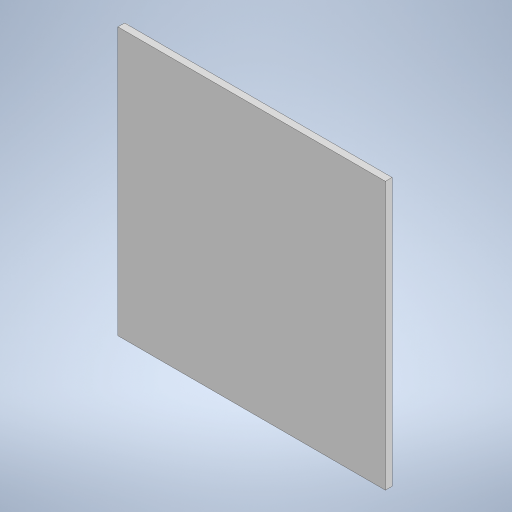
# Autodesk Inventor part: MLAtry1
Saved by Autodesk Inventor 2023 (Build 270158000, 158)
## iProperties
Created: 2022-05-28
Part Number: MLAtry1
Material: Generisch
Document SubType Name: Modeling
Designer: Tim Stechel
Density: 1 g/cm^3
Appearance: Vorgabe
Author: Tim Stechel
Autodesk Inventor part; units mm, degrees
(part 1 of 3)
ref_plane "YZ Plane" through (0, 0, 0) normal (1, 0, 0) x (0, 1, 0)
ref_plane "XZ Plane" through (0, 0, 0) normal (0, 1, 0) x (-1, 0, 0)
ref_plane "XY Plane" through (0, 0, 0) normal (0, 0, 1) x (1, 0, 0)
sketch "Skizze1" plane through (0, 0, 0) normal (0, 0, 1) x (1, 0, 0)
  line L0 (-10, 10) -> (10, 10)
  line L1 (10, 10) -> (10, -10)
  line L2 (10, -10) -> (-10, -10)
  line L3 (-10, -10) -> (-10, 10)
  line L4 (0, -4.8324) -> (0, 6.8811)
  line L5 (-11.9742, 0) -> (8.646, 0)
  line L6 (-10, 10) -> (-10, 9.85)
  line L7 (-10, 9.85) -> (10, 9.85)
  line L8 (-10, 10) -> (-9.85, 10)
  line L9 (-9.85, 10) -> (-9.85, -10)
  circle A0 centre (-9.85, 9.85) radius 0.15
  line L10 (-10, 10) -> (10, 10)
  line L11 (10, 10) -> (10, -10)
  line L12 (10, -10) -> (-10, -10)
  line L13 (-10, -10) -> (-10, 10)
  circle A1 centre (-9.85, 9.55) radius 0.15
  circle A2 centre (-9.85, 9.25) radius 0.15
  circle A3 centre (-9.85, 8.95) radius 0.15
  circle A4 centre (-9.85, 8.65) radius 0.15
  circle A5 centre (-9.85, 8.35) radius 0.15
  circle A6 centre (-9.85, 8.05) radius 0.15
  circle A7 centre (-9.85, 7.75) radius 0.15
  circle A8 centre (-9.85, 7.45) radius 0.15
  circle A9 centre (-9.85, 7.15) radius 0.15
  circle A10 centre (-9.85, 6.85) radius 0.15
  circle A11 centre (-9.85, 6.55) radius 0.15
  circle A12 centre (-9.85, 6.25) radius 0.15
  circle A13 centre (-9.85, 5.95) radius 0.15
  circle A14 centre (-9.85, 5.65) radius 0.15
  circle A15 centre (-9.85, 5.35) radius 0.15
  circle A16 centre (-9.85, 5.05) radius 0.15
  circle A17 centre (-9.85, 4.75) radius 0.15
  circle A18 centre (-9.85, 4.45) radius 0.15
  circle A19 centre (-9.85, 4.15) radius 0.15
  circle A20 centre (-9.85, 3.85) radius 0.15
  circle A21 centre (-9.85, 3.55) radius 0.15
  circle A22 centre (-9.85, 3.25) radius 0.15
  circle A23 centre (-9.85, 2.95) radius 0.15
  circle A24 centre (-9.85, 2.65) radius 0.15
  circle A25 centre (-9.85, 2.35) radius 0.15
  circle A26 centre (-9.85, 2.05) radius 0.15
  circle A27 centre (-9.85, 1.75) radius 0.15
  circle A28 centre (-9.85, 1.45) radius 0.15
  circle A29 centre (-9.85, 1.15) radius 0.15
  circle A30 centre (-9.85, 0.85) radius 0.15
  circle A31 centre (-9.85, 0.55) radius 0.15
  circle A32 centre (-9.85, 0.25) radius 0.15
  circle A33 centre (-9.85, -0.05) radius 0.15
  circle A34 centre (-9.85, -0.35) radius 0.15
  circle A35 centre (-9.85, -0.65) radius 0.15
  circle A36 centre (-9.85, -0.95) radius 0.15
  circle A37 centre (-9.85, -1.25) radius 0.15
  circle A38 centre (-9.85, -1.55) radius 0.15
  circle A39 centre (-9.85, -1.85) radius 0.15
  circle A40 centre (-9.85, -2.15) radius 0.15
  circle A41 centre (-9.85, -2.45) radius 0.15
  circle A42 centre (-9.85, -2.75) radius 0.15
  circle A43 centre (-9.85, -3.05) radius 0.15
  circle A44 centre (-9.85, -3.35) radius 0.15
  circle A45 centre (-9.85, -3.65) radius 0.15
  circle A46 centre (-9.85, -3.95) radius 0.15
  circle A47 centre (-9.85, -4.25) radius 0.15
  circle A48 centre (-9.85, -4.55) radius 0.15
  circle A49 centre (-9.85, -4.85) radius 0.15
  circle A50 centre (-9.55, 9.85) radius 0.15
  circle A51 centre (-9.55, 9.55) radius 0.15
  circle A52 centre (-9.55, 9.25) radius 0.15
  circle A53 centre (-9.55, 8.95) radius 0.15
  circle A54 centre (-9.55, 8.65) radius 0.15
  circle A55 centre (-9.55, 8.35) radius 0.15
  circle A56 centre (-9.55, 8.05) radius 0.15
  circle A57 centre (-9.55, 7.75) radius 0.15
  circle A58 centre (-9.55, 7.45) radius 0.15
  circle A59 centre (-9.55, 7.15) radius 0.15
  circle A60 centre (-9.55, 6.85) radius 0.15
  circle A61 centre (-9.55, 6.55) radius 0.15
  circle A62 centre (-9.55, 6.25) radius 0.15
  circle A63 centre (-9.55, 5.95) radius 0.15
  circle A64 centre (-9.55, 5.65) radius 0.15
  circle A65 centre (-9.55, 5.35) radius 0.15
  circle A66 centre (-9.55, 5.05) radius 0.15
  circle A67 centre (-9.55, 4.75) radius 0.15
  circle A68 centre (-9.55, 4.45) radius 0.15
  circle A69 centre (-9.55, 4.15) radius 0.15
  circle A70 centre (-9.55, 3.85) radius 0.15
  circle A71 centre (-9.55, 3.55) radius 0.15
  circle A72 centre (-9.55, 3.25) radius 0.15
  circle A73 centre (-9.55, 2.95) radius 0.15
  circle A74 centre (-9.55, 2.65) radius 0.15
  circle A75 centre (-9.55, 2.35) radius 0.15
  circle A76 centre (-9.55, 2.05) radius 0.15
  circle A77 centre (-9.55, 1.75) radius 0.15
  circle A78 centre (-9.55, 1.45) radius 0.15
  circle A79 centre (-9.55, 1.15) radius 0.15
  circle A80 centre (-9.55, 0.85) radius 0.15
  circle A81 centre (-9.55, 0.55) radius 0.15
  circle A82 centre (-9.55, 0.25) radius 0.15
  circle A83 centre (-9.55, -0.05) radius 0.15
  circle A84 centre (-9.55, -0.35) radius 0.15
  circle A85 centre (-9.55, -0.65) radius 0.15
  circle A86 centre (-9.55, -0.95) radius 0.15
  circle A87 centre (-9.55, -1.25) radius 0.15
  circle A88 centre (-9.55, -1.55) radius 0.15
  circle A89 centre (-9.55, -1.85) radius 0.15
  circle A90 centre (-9.55, -2.15) radius 0.15
  circle A91 centre (-9.55, -2.45) radius 0.15
  circle A92 centre (-9.55, -2.75) radius 0.15
  circle A93 centre (-9.55, -3.05) radius 0.15
  circle A94 centre (-9.55, -3.35) radius 0.15
  circle A95 centre (-9.55, -3.65) radius 0.15
  circle A96 centre (-9.55, -3.95) radius 0.15
  circle A97 centre (-9.55, -4.25) radius 0.15
  circle A98 centre (-9.55, -4.55) radius 0.15
  circle A99 centre (-9.55, -4.85) radius 0.15
  circle A100 centre (-9.25, 9.85) radius 0.15
  circle A101 centre (-9.25, 9.55) radius 0.15
  circle A102 centre (-9.25, 9.25) radius 0.15
  circle A103 centre (-9.25, 8.95) radius 0.15
  circle A104 centre (-9.25, 8.65) radius 0.15
  circle A105 centre (-9.25, 8.35) radius 0.15
  circle A106 centre (-9.25, 8.05) radius 0.15
  circle A107 centre (-9.25, 7.75) radius 0.15
  circle A108 centre (-9.25, 7.45) radius 0.15
  circle A109 centre (-9.25, 7.15) radius 0.15
  circle A110 centre (-9.25, 6.85) radius 0.15
  circle A111 centre (-9.25, 6.55) radius 0.15
  circle A112 centre (-9.25, 6.25) radius 0.15
  circle A113 centre (-9.25, 5.95) radius 0.15
  circle A114 centre (-9.25, 5.65) radius 0.15
  circle A115 centre (-9.25, 5.35) radius 0.15
  circle A116 centre (-9.25, 5.05) radius 0.15
  circle A117 centre (-9.25, 4.75) radius 0.15
  circle A118 centre (-9.25, 4.45) radius 0.15
  circle A119 centre (-9.25, 4.15) radius 0.15
  circle A120 centre (-9.25, 3.85) radius 0.15
  circle A121 centre (-9.25, 3.55) radius 0.15
  circle A122 centre (-9.25, 3.25) radius 0.15
  circle A123 centre (-9.25, 2.95) radius 0.15
  circle A124 centre (-9.25, 2.65) radius 0.15
  circle A125 centre (-9.25, 2.35) radius 0.15
  circle A126 centre (-9.25, 2.05) radius 0.15
  circle A127 centre (-9.25, 1.75) radius 0.15
  circle A128 centre (-9.25, 1.45) radius 0.15
  circle A129 centre (-9.25, 1.15) radius 0.15
  circle A130 centre (-9.25, 0.85) radius 0.15
  circle A131 centre (-9.25, 0.55) radius 0.15
  circle A132 centre (-9.25, 0.25) radius 0.15
  circle A133 centre (-9.25, -0.05) radius 0.15
  circle A134 centre (-9.25, -0.35) radius 0.15
  circle A135 centre (-9.25, -0.65) radius 0.15
  circle A136 centre (-9.25, -0.95) radius 0.15
  circle A137 centre (-9.25, -1.25) radius 0.15
  circle A138 centre (-9.25, -1.55) radius 0.15
  circle A139 centre (-9.25, -1.85) radius 0.15
  circle A140 centre (-9.25, -2.15) radius 0.15
  circle A141 centre (-9.25, -2.45) radius 0.15
  circle A142 centre (-9.25, -2.75) radius 0.15
  circle A143 centre (-9.25, -3.05) radius 0.15
  circle A144 centre (-9.25, -3.35) radius 0.15
  circle A145 centre (-9.25, -3.65) radius 0.15
  circle A146 centre (-9.25, -3.95) radius 0.15
  circle A147 centre (-9.25, -4.25) radius 0.15
  circle A148 centre (-9.25, -4.55) radius 0.15
  circle A149 centre (-9.25, -4.85) radius 0.15
  circle A150 centre (-8.95, 9.85) radius 0.15
  circle A151 centre (-8.95, 9.55) radius 0.15
  circle A152 centre (-8.95, 9.25) radius 0.15
  circle A153 centre (-8.95, 8.95) radius 0.15
  circle A154 centre (-8.95, 8.65) radius 0.15
  circle A155 centre (-8.95, 8.35) radius 0.15
  circle A156 centre (-8.95, 8.05) radius 0.15
  circle A157 centre (-8.95, 7.75) radius 0.15
  circle A158 centre (-8.95, 7.45) radius 0.15
  circle A159 centre (-8.95, 7.15) radius 0.15
  circle A160 centre (-8.95, 6.85) radius 0.15
  circle A161 centre (-8.95, 6.55) radius 0.15
  circle A162 centre (-8.95, 6.25) radius 0.15
  circle A163 centre (-8.95, 5.95) radius 0.15
  circle A164 centre (-8.95, 5.65) radius 0.15
  circle A165 centre (-8.95, 5.35) radius 0.15
  circle A166 centre (-8.95, 5.05) radius 0.15
  circle A167 centre (-8.95, 4.75) radius 0.15
  circle A168 centre (-8.95, 4.45) radius 0.15
  circle A169 centre (-8.95, 4.15) radius 0.15
  circle A170 centre (-8.95, 3.85) radius 0.15
  circle A171 centre (-8.95, 3.55) radius 0.15
  circle A172 centre (-8.95, 3.25) radius 0.15
  circle A173 centre (-8.95, 2.95) radius 0.15
  circle A174 centre (-8.95, 2.65) radius 0.15
  circle A175 centre (-8.95, 2.35) radius 0.15
  circle A176 centre (-8.95, 2.05) radius 0.15
  circle A177 centre (-8.95, 1.75) radius 0.15
  circle A178 centre (-8.95, 1.45) radius 0.15
  circle A179 centre (-8.95, 1.15) radius 0.15
  circle A180 centre (-8.95, 0.85) radius 0.15
  circle A181 centre (-8.95, 0.55) radius 0.15
  circle A182 centre (-8.95, 0.25) radius 0.15
  circle A183 centre (-8.95, -0.05) radius 0.15
  circle A184 centre (-8.95, -0.35) radius 0.15
  circle A185 centre (-8.95, -0.65) radius 0.15
  circle A186 centre (-8.95, -0.95) radius 0.15
  circle A187 centre (-8.95, -1.25) radius 0.15
  circle A188 centre (-8.95, -1.55) radius 0.15
  circle A189 centre (-8.95, -1.85) radius 0.15
  circle A190 centre (-8.95, -2.15) radius 0.15
  circle A191 centre (-8.95, -2.45) radius 0.15
  circle A192 centre (-8.95, -2.75) radius 0.15
  circle A193 centre (-8.95, -3.05) radius 0.15
  circle A194 centre (-8.95, -3.35) radius 0.15
  circle A195 centre (-8.95, -3.65) radius 0.15
  circle A196 centre (-8.95, -3.95) radius 0.15
  circle A197 centre (-8.95, -4.25) radius 0.15
  circle A198 centre (-8.95, -4.55) radius 0.15
  circle A199 centre (-8.95, -4.85) radius 0.15
  circle A200 centre (-8.65, 9.85) radius 0.15
  circle A201 centre (-8.65, 9.55) radius 0.15
  circle A202 centre (-8.65, 9.25) radius 0.15
  circle A203 centre (-8.65, 8.95) radius 0.15
  circle A204 centre (-8.65, 8.65) radius 0.15
  circle A205 centre (-8.65, 8.35) radius 0.15
  circle A206 centre (-8.65, 8.05) radius 0.15
  circle A207 centre (-8.65, 7.75) radius 0.15
  circle A208 centre (-8.65, 7.45) radius 0.15
  circle A209 centre (-8.65, 7.15) radius 0.15
  circle A210 centre (-8.65, 6.85) radius 0.15
  circle A211 centre (-8.65, 6.55) radius 0.15
  circle A212 centre (-8.65, 6.25) radius 0.15
  circle A213 centre (-8.65, 5.95) radius 0.15
  circle A214 centre (-8.65, 5.65) radius 0.15
  circle A215 centre (-8.65, 5.35) radius 0.15
  circle A216 centre (-8.65, 5.05) radius 0.15
  circle A217 centre (-8.65, 4.75) radius 0.15
  circle A218 centre (-8.65, 4.45) radius 0.15
  circle A219 centre (-8.65, 4.15) radius 0.15
  circle A220 centre (-8.65, 3.85) radius 0.15
  circle A221 centre (-8.65, 3.55) radius 0.15
  circle A222 centre (-8.65, 3.25) radius 0.15
  circle A223 centre (-8.65, 2.95) radius 0.15
  circle A224 centre (-8.65, 2.65) radius 0.15
  circle A225 centre (-8.65, 2.35) radius 0.15
  circle A226 centre (-8.65, 2.05) radius 0.15
  circle A227 centre (-8.65, 1.75) radius 0.15
  circle A228 centre (-8.65, 1.45) radius 0.15
  circle A229 centre (-8.65, 1.15) radius 0.15
  circle A230 centre (-8.65, 0.85) radius 0.15
  circle A231 centre (-8.65, 0.55) radius 0.15
  circle A232 centre (-8.65, 0.25) radius 0.15
  circle A233 centre (-8.65, -0.05) radius 0.15
  circle A234 centre (-8.65, -0.35) radius 0.15
  circle A235 centre (-8.65, -0.65) radius 0.15
  circle A236 centre (-8.65, -0.95) radius 0.15
  circle A237 centre (-8.65, -1.25) radius 0.15
  circle A238 centre (-8.65, -1.55) radius 0.15
  circle A239 centre (-8.65, -1.85) radius 0.15
  circle A240 centre (-8.65, -2.15) radius 0.15
  circle A241 centre (-8.65, -2.45) radius 0.15
  circle A242 centre (-8.65, -2.75) radius 0.15
  circle A243 centre (-8.65, -3.05) radius 0.15
  circle A244 centre (-8.65, -3.35) radius 0.15
  circle A245 centre (-8.65, -3.65) radius 0.15
  circle A246 centre (-8.65, -3.95) radius 0.15
  circle A247 centre (-8.65, -4.25) radius 0.15
  circle A248 centre (-8.65, -4.55) radius 0.15
  circle A249 centre (-8.65, -4.85) radius 0.15
  circle A250 centre (-8.35, 9.85) radius 0.15
  circle A251 centre (-8.35, 9.55) radius 0.15
  circle A252 centre (-8.35, 9.25) radius 0.15
  circle A253 centre (-8.35, 8.95) radius 0.15
  circle A254 centre (-8.35, 8.65) radius 0.15
  circle A255 centre (-8.35, 8.35) radius 0.15
  circle A256 centre (-8.35, 8.05) radius 0.15
  circle A257 centre (-8.35, 7.75) radius 0.15
  circle A258 centre (-8.35, 7.45) radius 0.15
  circle A259 centre (-8.35, 7.15) radius 0.15
  circle A260 centre (-8.35, 6.85) radius 0.15
  circle A261 centre (-8.35, 6.55) radius 0.15
  circle A262 centre (-8.35, 6.25) radius 0.15
  circle A263 centre (-8.35, 5.95) radius 0.15
  circle A264 centre (-8.35, 5.65) radius 0.15
  circle A265 centre (-8.35, 5.35) radius 0.15
  circle A266 centre (-8.35, 5.05) radius 0.15
  circle A267 centre (-8.35, 4.75) radius 0.15
  circle A268 centre (-8.35, 4.45) radius 0.15
  circle A269 centre (-8.35, 4.15) radius 0.15
  circle A270 centre (-8.35, 3.85) radius 0.15
  circle A271 centre (-8.35, 3.55) radius 0.15
  circle A272 centre (-8.35, 3.25) radius 0.15
  circle A273 centre (-8.35, 2.95) radius 0.15
  circle A274 centre (-8.35, 2.65) radius 0.15
  circle A275 centre (-8.35, 2.35) radius 0.15
  circle A276 centre (-8.35, 2.05) radius 0.15
  circle A277 centre (-8.35, 1.75) radius 0.15
  circle A278 centre (-8.35, 1.45) radius 0.15
  circle A279 centre (-8.35, 1.15) radius 0.15
  circle A280 centre (-8.35, 0.85) radius 0.15
  circle A281 centre (-8.35, 0.55) radius 0.15
  circle A282 centre (-8.35, 0.25) radius 0.15
  circle A283 centre (-8.35, -0.05) radius 0.15
  circle A284 centre (-8.35, -0.35) radius 0.15
  circle A285 centre (-8.35, -0.65) radius 0.15
  circle A286 centre (-8.35, -0.95) radius 0.15
  circle A287 centre (-8.35, -1.25) radius 0.15
  circle A288 centre (-8.35, -1.55) radius 0.15
  circle A289 centre (-8.35, -1.85) radius 0.15
  circle A290 centre (-8.35, -2.15) radius 0.15
  circle A291 centre (-8.35, -2.45) radius 0.15
  circle A292 centre (-8.35, -2.75) radius 0.15
  circle A293 centre (-8.35, -3.05) radius 0.15
  circle A294 centre (-8.35, -3.35) radius 0.15
  circle A295 centre (-8.35, -3.65) radius 0.15
  circle A296 centre (-8.35, -3.95) radius 0.15
  circle A297 centre (-8.35, -4.25) radius 0.15
  circle A298 centre (-8.35, -4.55) radius 0.15
  circle A299 centre (-8.35, -4.85) radius 0.15
  circle A300 centre (-8.05, 9.85) radius 0.15
  circle A301 centre (-8.05, 9.55) radius 0.15
  circle A302 centre (-8.05, 9.25) radius 0.15
  circle A303 centre (-8.05, 8.95) radius 0.15
  circle A304 centre (-8.05, 8.65) radius 0.15
  circle A305 centre (-8.05, 8.35) radius 0.15
  circle A306 centre (-8.05, 8.05) radius 0.15
  circle A307 centre (-8.05, 7.75) radius 0.15
  circle A308 centre (-8.05, 7.45) radius 0.15
  circle A309 centre (-8.05, 7.15) radius 0.15
  circle A310 centre (-8.05, 6.85) radius 0.15
  circle A311 centre (-8.05, 6.55) radius 0.15
  circle A312 centre (-8.05, 6.25) radius 0.15
  circle A313 centre (-8.05, 5.95) radius 0.15
  circle A314 centre (-8.05, 5.65) radius 0.15
  circle A315 centre (-8.05, 5.35) radius 0.15
  circle A316 centre (-8.05, 5.05) radius 0.15
  circle A317 centre (-8.05, 4.75) radius 0.15
  circle A318 centre (-8.05, 4.45) radius 0.15
  circle A319 centre (-8.05, 4.15) radius 0.15
  circle A320 centre (-8.05, 3.85) radius 0.15
  circle A321 centre (-8.05, 3.55) radius 0.15
  circle A322 centre (-8.05, 3.25) radius 0.15
  circle A323 centre (-8.05, 2.95) radius 0.15
  circle A324 centre (-8.05, 2.65) radius 0.15
  circle A325 centre (-8.05, 2.35) radius 0.15
  circle A326 centre (-8.05, 2.05) radius 0.15
  circle A327 centre (-8.05, 1.75) radius 0.15
  circle A328 centre (-8.05, 1.45) radius 0.15
  circle A329 centre (-8.05, 1.15) radius 0.15
  circle A330 centre (-8.05, 0.85) radius 0.15
  circle A331 centre (-8.05, 0.55) radius 0.15
  circle A332 centre (-8.05, 0.25) radius 0.15
  circle A333 centre (-8.05, -0.05) radius 0.15
  circle A334 centre (-8.05, -0.35) radius 0.15
  circle A335 centre (-8.05, -0.65) radius 0.15
  circle A336 centre (-8.05, -0.95) radius 0.15
  circle A337 centre (-8.05, -1.25) radius 0.15
  circle A338 centre (-8.05, -1.55) radius 0.15
  circle A339 centre (-8.05, -1.85) radius 0.15
  circle A340 centre (-8.05, -2.15) radius 0.15
  circle A341 centre (-8.05, -2.45) radius 0.15
  circle A342 centre (-8.05, -2.75) radius 0.15
  circle A343 centre (-8.05, -3.05) radius 0.15
  circle A344 centre (-8.05, -3.35) radius 0.15
  circle A345 centre (-8.05, -3.65) radius 0.15
  circle A346 centre (-8.05, -3.95) radius 0.15
  circle A347 centre (-8.05, -4.25) radius 0.15
  circle A348 centre (-8.05, -4.55) radius 0.15
  circle A349 centre (-8.05, -4.85) radius 0.15
  circle A350 centre (-7.75, 9.85) radius 0.15
  circle A351 centre (-7.75, 9.55) radius 0.15
  circle A352 centre (-7.75, 9.25) radius 0.15
  circle A353 centre (-7.75, 8.95) radius 0.15
  circle A354 centre (-7.75, 8.65) radius 0.15
  circle A355 centre (-7.75, 8.35) radius 0.15
  circle A356 centre (-7.75, 8.05) radius 0.15
  circle A357 centre (-7.75, 7.75) radius 0.15
  circle A358 centre (-7.75, 7.45) radius 0.15
  circle A359 centre (-7.75, 7.15) radius 0.15
  circle A360 centre (-7.75, 6.85) radius 0.15
  circle A361 centre (-7.75, 6.55) radius 0.15
  circle A362 centre (-7.75, 6.25) radius 0.15
  circle A363 centre (-7.75, 5.95) radius 0.15
  circle A364 centre (-7.75, 5.65) radius 0.15
  circle A365 centre (-7.75, 5.35) radius 0.15
  circle A366 centre (-7.75, 5.05) radius 0.15
  circle A367 centre (-7.75, 4.75) radius 0.15
  circle A368 centre (-7.75, 4.45) radius 0.15
  circle A369 centre (-7.75, 4.15) radius 0.15
  circle A370 centre (-7.75, 3.85) radius 0.15
  circle A371 centre (-7.75, 3.55) radius 0.15
  circle A372 centre (-7.75, 3.25) radius 0.15
  circle A373 centre (-7.75, 2.95) radius 0.15
  circle A374 centre (-7.75, 2.65) radius 0.15
  circle A375 centre (-7.75, 2.35) radius 0.15
  circle A376 centre (-7.75, 2.05) radius 0.15
  circle A377 centre (-7.75, 1.75) radius 0.15
  circle A378 centre (-7.75, 1.45) radius 0.15
  circle A379 centre (-7.75, 1.15) radius 0.15
  circle A380 centre (-7.75, 0.85) radius 0.15
  circle A381 centre (-7.75, 0.55) radius 0.15
  circle A382 centre (-7.75, 0.25) radius 0.15
  circle A383 centre (-7.75, -0.05) radius 0.15
  circle A384 centre (-7.75, -0.35) radius 0.15
  circle A385 centre (-7.75, -0.65) radius 0.15
  circle A386 centre (-7.75, -0.95) radius 0.15
  circle A387 centre (-7.75, -1.25) radius 0.15
  circle A388 centre (-7.75, -1.55) radius 0.15
  circle A389 centre (-7.75, -1.85) radius 0.15
  circle A390 centre (-7.75, -2.15) radius 0.15
  circle A391 centre (-7.75, -2.45) radius 0.15
  circle A392 centre (-7.75, -2.75) radius 0.15
  circle A393 centre (-7.75, -3.05) radius 0.15
  circle A394 centre (-7.75, -3.35) radius 0.15
  circle A395 centre (-7.75, -3.65) radius 0.15
  circle A396 centre (-7.75, -3.95) radius 0.15
  circle A397 centre (-7.75, -4.25) radius 0.15
  circle A398 centre (-7.75, -4.55) radius 0.15
  circle A399 centre (-7.75, -4.85) radius 0.15
  circle A400 centre (-7.45, 9.85) radius 0.15
  circle A401 centre (-7.45, 9.55) radius 0.15
  circle A402 centre (-7.45, 9.25) radius 0.15
  circle A403 centre (-7.45, 8.95) radius 0.15
  circle A404 centre (-7.45, 8.65) radius 0.15
  circle A405 centre (-7.45, 8.35) radius 0.15
  circle A406 centre (-7.45, 8.05) radius 0.15
  circle A407 centre (-7.45, 7.75) radius 0.15
  circle A408 centre (-7.45, 7.45) radius 0.15
  circle A409 centre (-7.45, 7.15) radius 0.15
  circle A410 centre (-7.45, 6.85) radius 0.15
  circle A411 centre (-7.45, 6.55) radius 0.15
  circle A412 centre (-7.45, 6.25) radius 0.15
  circle A413 centre (-7.45, 5.95) radius 0.15
  circle A414 centre (-7.45, 5.65) radius 0.15
  circle A415 centre (-7.45, 5.35) radius 0.15
  circle A416 centre (-7.45, 5.05) radius 0.15
  circle A417 centre (-7.45, 4.75) radius 0.15
  circle A418 centre (-7.45, 4.45) radius 0.15
  circle A419 centre (-7.45, 4.15) radius 0.15
  circle A420 centre (-7.45, 3.85) radius 0.15
  circle A421 centre (-7.45, 3.55) radius 0.15
  circle A422 centre (-7.45, 3.25) radius 0.15
  circle A423 centre (-7.45, 2.95) radius 0.15
  circle A424 centre (-7.45, 2.65) radius 0.15
  circle A425 centre (-7.45, 2.35) radius 0.15
  circle A426 centre (-7.45, 2.05) radius 0.15
  circle A427 centre (-7.45, 1.75) radius 0.15
  circle A428 centre (-7.45, 1.45) radius 0.15
  circle A429 centre (-7.45, 1.15) radius 0.15
  circle A430 centre (-7.45, 0.85) radius 0.15
  circle A431 centre (-7.45, 0.55) radius 0.15
  circle A432 centre (-7.45, 0.25) radius 0.15
  circle A433 centre (-7.45, -0.05) radius 0.15
  circle A434 centre (-7.45, -0.35) radius 0.15
  circle A435 centre (-7.45, -0.65) radius 0.15
  circle A436 centre (-7.45, -0.95) radius 0.15
  circle A437 centre (-7.45, -1.25) radius 0.15
  circle A438 centre (-7.45, -1.55) radius 0.15
  circle A439 centre (-7.45, -1.85) radius 0.15
  circle A440 centre (-7.45, -2.15) radius 0.15
  circle A441 centre (-7.45, -2.45) radius 0.15
  circle A442 centre (-7.45, -2.75) radius 0.15
  circle A443 centre (-7.45, -3.05) radius 0.15
  circle A444 centre (-7.45, -3.35) radius 0.15
  circle A445 centre (-7.45, -3.65) radius 0.15
  circle A446 centre (-7.45, -3.95) radius 0.15
  circle A447 centre (-7.45, -4.25) radius 0.15
  circle A448 centre (-7.45, -4.55) radius 0.15
  circle A449 centre (-7.45, -4.85) radius 0.15
  circle A450 centre (-7.15, 9.85) radius 0.15
  circle A451 centre (-7.15, 9.55) radius 0.15
  circle A452 centre (-7.15, 9.25) radius 0.15
  circle A453 centre (-7.15, 8.95) radius 0.15
  circle A454 centre (-7.15, 8.65) radius 0.15
  circle A455 centre (-7.15, 8.35) radius 0.15
  circle A456 centre (-7.15, 8.05) radius 0.15
  circle A457 centre (-7.15, 7.75) radius 0.15
  circle A458 centre (-7.15, 7.45) radius 0.15
  circle A459 centre (-7.15, 7.15) radius 0.15
  circle A460 centre (-7.15, 6.85) radius 0.15
  circle A461 centre (-7.15, 6.55) radius 0.15
  circle A462 centre (-7.15, 6.25) radius 0.15
  circle A463 centre (-7.15, 5.95) radius 0.15
  circle A464 centre (-7.15, 5.65) radius 0.15
  circle A465 centre (-7.15, 5.35) radius 0.15
  circle A466 centre (-7.15, 5.05) radius 0.15
  circle A467 centre (-7.15, 4.75) radius 0.15
  circle A468 centre (-7.15, 4.45) radius 0.15
  circle A469 centre (-7.15, 4.15) radius 0.15
  circle A470 centre (-7.15, 3.85) radius 0.15
  circle A471 centre (-7.15, 3.55) radius 0.15
  circle A472 centre (-7.15, 3.25) radius 0.15
  circle A473 centre (-7.15, 2.95) radius 0.15
  circle A474 centre (-7.15, 2.65) radius 0.15
  circle A475 centre (-7.15, 2.35) radius 0.15
  circle A476 centre (-7.15, 2.05) radius 0.15
  circle A477 centre (-7.15, 1.75) radius 0.15
  circle A478 centre (-7.15, 1.45) radius 0.15
  circle A479 centre (-7.15, 1.15) radius 0.15
  circle A480 centre (-7.15, 0.85) radius 0.15
  circle A481 centre (-7.15, 0.55) radius 0.15
  circle A482 centre (-7.15, 0.25) radius 0.15
  circle A483 centre (-7.15, -0.05) radius 0.15
  circle A484 centre (-7.15, -0.35) radius 0.15
  circle A485 centre (-7.15, -0.65) radius 0.15
  circle A486 centre (-7.15, -0.95) radius 0.15
  circle A487 centre (-7.15, -1.25) radius 0.15
  circle A488 centre (-7.15, -1.55) radius 0.15
  circle A489 centre (-7.15, -1.85) radius 0.15
  circle A490 centre (-7.15, -2.15) radius 0.15
  circle A491 centre (-7.15, -2.45) radius 0.15
  circle A492 centre (-7.15, -2.75) radius 0.15
  circle A493 centre (-7.15, -3.05) radius 0.15
  circle A494 centre (-7.15, -3.35) radius 0.15
  circle A495 centre (-7.15, -3.65) radius 0.15
  circle A496 centre (-7.15, -3.95) radius 0.15
  circle A497 centre (-7.15, -4.25) radius 0.15
  circle A498 centre (-7.15, -4.55) radius 0.15
  circle A499 centre (-7.15, -4.85) radius 0.15
  circle A500 centre (-6.85, 9.85) radius 0.15
  circle A501 centre (-6.85, 9.55) radius 0.15
  circle A502 centre (-6.85, 9.25) radius 0.15
  circle A503 centre (-6.85, 8.95) radius 0.15
  circle A504 centre (-6.85, 8.65) radius 0.15
  circle A505 centre (-6.85, 8.35) radius 0.15
  circle A506 centre (-6.85, 8.05) radius 0.15
  circle A507 centre (-6.85, 7.75) radius 0.15
  circle A508 centre (-6.85, 7.45) radius 0.15
  circle A509 centre (-6.85, 7.15) radius 0.15
  circle A510 centre (-6.85, 6.85) radius 0.15
  circle A511 centre (-6.85, 6.55) radius 0.15
  circle A512 centre (-6.85, 6.25) radius 0.15
  circle A513 centre (-6.85, 5.95) radius 0.15
  circle A514 centre (-6.85, 5.65) radius 0.15
  circle A515 centre (-6.85, 5.35) radius 0.15
  circle A516 centre (-6.85, 5.05) radius 0.15
  circle A517 centre (-6.85, 4.75) radius 0.15
  circle A518 centre (-6.85, 4.45) radius 0.15
  circle A519 centre (-6.85, 4.15) radius 0.15
  circle A520 centre (-6.85, 3.85) radius 0.15
  circle A521 centre (-6.85, 3.55) radius 0.15
  circle A522 centre (-6.85, 3.25) radius 0.15
  circle A523 centre (-6.85, 2.95) radius 0.15
  circle A524 centre (-6.85, 2.65) radius 0.15
  circle A525 centre (-6.85, 2.35) radius 0.15
  circle A526 centre (-6.85, 2.05) radius 0.15
  circle A527 centre (-6.85, 1.75) radius 0.15
  circle A528 centre (-6.85, 1.45) radius 0.15
  circle A529 centre (-6.85, 1.15) radius 0.15
  circle A530 centre (-6.85, 0.85) radius 0.15
  circle A531 centre (-6.85, 0.55) radius 0.15
  circle A532 centre (-6.85, 0.25) radius 0.15
  circle A533 centre (-6.85, -0.05) radius 0.15
  circle A534 centre (-6.85, -0.35) radius 0.15
  circle A535 centre (-6.85, -0.65) radius 0.15
  circle A536 centre (-6.85, -0.95) radius 0.15
  circle A537 centre (-6.85, -1.25) radius 0.15
  circle A538 centre (-6.85, -1.55) radius 0.15
  circle A539 centre (-6.85, -1.85) radius 0.15
  circle A540 centre (-6.85, -2.15) radius 0.15
  circle A541 centre (-6.85, -2.45) radius 0.15
  circle A542 centre (-6.85, -2.75) radius 0.15
  circle A543 centre (-6.85, -3.05) radius 0.15
  circle A544 centre (-6.85, -3.35) radius 0.15
  circle A545 centre (-6.85, -3.65) radius 0.15
  circle A546 centre (-6.85, -3.95) radius 0.15
  circle A547 centre (-6.85, -4.25) radius 0.15
  circle A548 centre (-6.85, -4.55) radius 0.15
  circle A549 centre (-6.85, -4.85) radius 0.15
  circle A550 centre (-6.55, 9.85) radius 0.15
  circle A551 centre (-6.55, 9.55) radius 0.15
  circle A552 centre (-6.55, 9.25) radius 0.15
  circle A553 centre (-6.55, 8.95) radius 0.15
  circle A554 centre (-6.55, 8.65) radius 0.15
  circle A555 centre (-6.55, 8.35) radius 0.15
  circle A556 centre (-6.55, 8.05) radius 0.15
  circle A557 centre (-6.55, 7.75) radius 0.15
  circle A558 centre (-6.55, 7.45) radius 0.15
  circle A559 centre (-6.55, 7.15) radius 0.15
  circle A560 centre (-6.55, 6.85) radius 0.15
  circle A561 centre (-6.55, 6.55) radius 0.15
  circle A562 centre (-6.55, 6.25) radius 0.15
  circle A563 centre (-6.55, 5.95) radius 0.15
  circle A564 centre (-6.55, 5.65) radius 0.15
  circle A565 centre (-6.55, 5.35) radius 0.15
  circle A566 centre (-6.55, 5.05) radius 0.15
  circle A567 centre (-6.55, 4.75) radius 0.15
  circle A568 centre (-6.55, 4.45) radius 0.15
  circle A569 centre (-6.55, 4.15) radius 0.15
  circle A570 centre (-6.55, 3.85) radius 0.15
  circle A571 centre (-6.55, 3.55) radius 0.15
  circle A572 centre (-6.55, 3.25) radius 0.15
  circle A573 centre (-6.55, 2.95) radius 0.15
  circle A574 centre (-6.55, 2.65) radius 0.15
  circle A575 centre (-6.55, 2.35) radius 0.15
  circle A576 centre (-6.55, 2.05) radius 0.15
  circle A577 centre (-6.55, 1.75) radius 0.15
  circle A578 centre (-6.55, 1.45) radius 0.15
  circle A579 centre (-6.55, 1.15) radius 0.15
  circle A580 centre (-6.55, 0.85) radius 0.15
  circle A581 centre (-6.55, 0.55) radius 0.15
  circle A582 centre (-6.55, 0.25) radius 0.15
  circle A583 centre (-6.55, -0.05) radius 0.15
  circle A584 centre (-6.55, -0.35) radius 0.15
  circle A585 centre (-6.55, -0.65) radius 0.15
  circle A586 centre (-6.55, -0.95) radius 0.15
  circle A587 centre (-6.55, -1.25) radius 0.15
  circle A588 centre (-6.55, -1.55) radius 0.15
  circle A589 centre (-6.55, -1.85) radius 0.15
  circle A590 centre (-6.55, -2.15) radius 0.15
  circle A591 centre (-6.55, -2.45) radius 0.15
  circle A592 centre (-6.55, -2.75) radius 0.15
  circle A593 centre (-6.55, -3.05) radius 0.15
  circle A594 centre (-6.55, -3.35) radius 0.15
  circle A595 centre (-6.55, -3.65) radius 0.15
  circle A596 centre (-6.55, -3.95) radius 0.15
  circle A597 centre (-6.55, -4.25) radius 0.15
  circle A598 centre (-6.55, -4.55) radius 0.15
  circle A599 centre (-6.55, -4.85) radius 0.15
  circle A600 centre (-6.25, 9.85) radius 0.15
  circle A601 centre (-6.25, 9.55) radius 0.15
  circle A602 centre (-6.25, 9.25) radius 0.15
  circle A603 centre (-6.25, 8.95) radius 0.15
  circle A604 centre (-6.25, 8.65) radius 0.15
  circle A605 centre (-6.25, 8.35) radius 0.15
  circle A606 centre (-6.25, 8.05) radius 0.15
  circle A607 centre (-6.25, 7.75) radius 0.15
  circle A608 centre (-6.25, 7.45) radius 0.15
  circle A609 centre (-6.25, 7.15) radius 0.15
  circle A610 centre (-6.25, 6.85) radius 0.15
  circle A611 centre (-6.25, 6.55) radius 0.15
  circle A612 centre (-6.25, 6.25) radius 0.15
  circle A613 centre (-6.25, 5.95) radius 0.15
  circle A614 centre (-6.25, 5.65) radius 0.15
  circle A615 centre (-6.25, 5.35) radius 0.15
  circle A616 centre (-6.25, 5.05) radius 0.15
  circle A617 centre (-6.25, 4.75) radius 0.15
  circle A618 centre (-6.25, 4.45) radius 0.15
  circle A619 centre (-6.25, 4.15) radius 0.15
  circle A620 centre (-6.25, 3.85) radius 0.15
  circle A621 centre (-6.25, 3.55) radius 0.15
  circle A622 centre (-6.25, 3.25) radius 0.15
  circle A623 centre (-6.25, 2.95) radius 0.15
  circle A624 centre (-6.25, 2.65) radius 0.15
  circle A625 centre (-6.25, 2.35) radius 0.15
  circle A626 centre (-6.25, 2.05) radius 0.15
  circle A627 centre (-6.25, 1.75) radius 0.15
  circle A628 centre (-6.25, 1.45) radius 0.15
  circle A629 centre (-6.25, 1.15) radius 0.15
  circle A630 centre (-6.25, 0.85) radius 0.15
  circle A631 centre (-6.25, 0.55) radius 0.15
  circle A632 centre (-6.25, 0.25) radius 0.15
  circle A633 centre (-6.25, -0.05) radius 0.15
  circle A634 centre (-6.25, -0.35) radius 0.15
  circle A635 centre (-6.25, -0.65) radius 0.15
  circle A636 centre (-6.25, -0.95) radius 0.15
  circle A637 centre (-6.25, -1.25) radius 0.15
  circle A638 centre (-6.25, -1.55) radius 0.15
  circle A639 centre (-6.25, -1.85) radius 0.15
  circle A640 centre (-6.25, -2.15) radius 0.15
  circle A641 centre (-6.25, -2.45) radius 0.15
  circle A642 centre (-6.25, -2.75) radius 0.15
  circle A643 centre (-6.25, -3.05) radius 0.15
  circle A644 centre (-6.25, -3.35) radius 0.15
  circle A645 centre (-6.25, -3.65) radius 0.15
  circle A646 centre (-6.25, -3.95) radius 0.15
  circle A647 centre (-6.25, -4.25) radius 0.15
  circle A648 centre (-6.25, -4.55) radius 0.15
  circle A649 centre (-6.25, -4.85) radius 0.15
  circle A650 centre (-5.95, 9.85) radius 0.15
  circle A651 centre (-5.95, 9.55) radius 0.15
  circle A652 centre (-5.95, 9.25) radius 0.15
  circle A653 centre (-5.95, 8.95) radius 0.15
  circle A654 centre (-5.95, 8.65) radius 0.15
  circle A655 centre (-5.95, 8.35) radius 0.15
  circle A656 centre (-5.95, 8.05) radius 0.15
  circle A657 centre (-5.95, 7.75) radius 0.15
  circle A658 centre (-5.95, 7.45) radius 0.15
  circle A659 centre (-5.95, 7.15) radius 0.15
  circle A660 centre (-5.95, 6.85) radius 0.15
  circle A661 centre (-5.95, 6.55) radius 0.15
  circle A662 centre (-5.95, 6.25) radius 0.15
  circle A663 centre (-5.95, 5.95) radius 0.15
  circle A664 centre (-5.95, 5.65) radius 0.15
  circle A665 centre (-5.95, 5.35) radius 0.15
  circle A666 centre (-5.95, 5.05) radius 0.15
  circle A667 centre (-5.95, 4.75) radius 0.15
  circle A668 centre (-5.95, 4.45) radius 0.15
  circle A669 centre (-5.95, 4.15) radius 0.15
  circle A670 centre (-5.95, 3.85) radius 0.15
  circle A671 centre (-5.95, 3.55) radius 0.15
  circle A672 centre (-5.95, 3.25) radius 0.15
  circle A673 centre (-5.95, 2.95) radius 0.15
  circle A674 centre (-5.95, 2.65) radius 0.15
  circle A675 centre (-5.95, 2.35) radius 0.15
  circle A676 centre (-5.95, 2.05) radius 0.15
  circle A677 centre (-5.95, 1.75) radius 0.15
  circle A678 centre (-5.95, 1.45) radius 0.15
  circle A679 centre (-5.95, 1.15) radius 0.15
  circle A680 centre (-5.95, 0.85) radius 0.15
  circle A681 centre (-5.95, 0.55) radius 0.15
  circle A682 centre (-5.95, 0.25) radius 0.15
  circle A683 centre (-5.95, -0.05) radius 0.15
  circle A684 centre (-5.95, -0.35) radius 0.15
  circle A685 centre (-5.95, -0.65) radius 0.15
  circle A686 centre (-5.95, -0.95) radius 0.15
  circle A687 centre (-5.95, -1.25) radius 0.15
  circle A688 centre (-5.95, -1.55) radius 0.15
  circle A689 centre (-5.95, -1.85) radius 0.15
  circle A690 centre (-5.95, -2.15) radius 0.15
  circle A691 centre (-5.95, -2.45) radius 0.15
  circle A692 centre (-5.95, -2.75) radius 0.15
  circle A693 centre (-5.95, -3.05) radius 0.15
  circle A694 centre (-5.95, -3.35) radius 0.15
  circle A695 centre (-5.95, -3.65) radius 0.15
  circle A696 centre (-5.95, -3.95) radius 0.15
  circle A697 centre (-5.95, -4.25) radius 0.15
  circle A698 centre (-5.95, -4.55) radius 0.15
  circle A699 centre (-5.95, -4.85) radius 0.15
  circle A700 centre (-5.65, 9.85) radius 0.15
  circle A701 centre (-5.65, 9.55) radius 0.15
  circle A702 centre (-5.65, 9.25) radius 0.15
  circle A703 centre (-5.65, 8.95) radius 0.15
  circle A704 centre (-5.65, 8.65) radius 0.15
  circle A705 centre (-5.65, 8.35) radius 0.15
  circle A706 centre (-5.65, 8.05) radius 0.15
  circle A707 centre (-5.65, 7.75) radius 0.15
  circle A708 centre (-5.65, 7.45) radius 0.15
  circle A709 centre (-5.65, 7.15) radius 0.15
  circle A710 centre (-5.65, 6.85) radius 0.15
  circle A711 centre (-5.65, 6.55) radius 0.15
  circle A712 centre (-5.65, 6.25) radius 0.15
  circle A713 centre (-5.65, 5.95) radius 0.15
  circle A714 centre (-5.65, 5.65) radius 0.15
  circle A715 centre (-5.65, 5.35) radius 0.15
  circle A716 centre (-5.65, 5.05) radius 0.15
  circle A717 centre (-5.65, 4.75) radius 0.15
  circle A718 centre (-5.65, 4.45) radius 0.15
  circle A719 centre (-5.65, 4.15) radius 0.15
  circle A720 centre (-5.65, 3.85) radius 0.15
  circle A721 centre (-5.65, 3.55) radius 0.15
  circle A722 centre (-5.65, 3.25) radius 0.15
  circle A723 centre (-5.65, 2.95) radius 0.15
  circle A724 centre (-5.65, 2.65) radius 0.15
  circle A725 centre (-5.65, 2.35) radius 0.15
  circle A726 centre (-5.65, 2.05) radius 0.15
  circle A727 centre (-5.65, 1.75) radius 0.15
  circle A728 centre (-5.65, 1.45) radius 0.15
  circle A729 centre (-5.65, 1.15) radius 0.15
  circle A730 centre (-5.65, 0.85) radius 0.15
  circle A731 centre (-5.65, 0.55) radius 0.15
  circle A732 centre (-5.65, 0.25) radius 0.15
  circle A733 centre (-5.65, -0.05) radius 0.15
  circle A734 centre (-5.65, -0.35) radius 0.15
  circle A735 centre (-5.65, -0.65) radius 0.15
  circle A736 centre (-5.65, -0.95) radius 0.15
  circle A737 centre (-5.65, -1.25) radius 0.15
  circle A738 centre (-5.65, -1.55) radius 0.15
  circle A739 centre (-5.65, -1.85) radius 0.15
  circle A740 centre (-5.65, -2.15) radius 0.15
  circle A741 centre (-5.65, -2.45) radius 0.15
  circle A742 centre (-5.65, -2.75) radius 0.15
  circle A743 centre (-5.65, -3.05) radius 0.15
  circle A744 centre (-5.65, -3.35) radius 0.15
  circle A745 centre (-5.65, -3.65) radius 0.15
  circle A746 centre (-5.65, -3.95) radius 0.15
  circle A747 centre (-5.65, -4.25) radius 0.15
  circle A748 centre (-5.65, -4.55) radius 0.15
  circle A749 centre (-5.65, -4.85) radius 0.15
  circle A750 centre (-5.35, 9.85) radius 0.15
  circle A751 centre (-5.35, 9.55) radius 0.15
  circle A752 centre (-5.35, 9.25) radius 0.15
  circle A753 centre (-5.35, 8.95) radius 0.15
  circle A754 centre (-5.35, 8.65) radius 0.15
  circle A755 centre (-5.35, 8.35) radius 0.15
  circle A756 centre (-5.35, 8.05) radius 0.15
  circle A757 centre (-5.35, 7.75) radius 0.15
  circle A758 centre (-5.35, 7.45) radius 0.15
  circle A759 centre (-5.35, 7.15) radius 0.15
  circle A760 centre (-5.35, 6.85) radius 0.15
  circle A761 centre (-5.35, 6.55) radius 0.15
  circle A762 centre (-5.35, 6.25) radius 0.15
  circle A763 centre (-5.35, 5.95) radius 0.15
  circle A764 centre (-5.35, 5.65) radius 0.15
  circle A765 centre (-5.35, 5.35) radius 0.15
  circle A766 centre (-5.35, 5.05) radius 0.15
  circle A767 centre (-5.35, 4.75) radius 0.15
  circle A768 centre (-5.35, 4.45) radius 0.15
  circle A769 centre (-5.35, 4.15) radius 0.15
  circle A770 centre (-5.35, 3.85) radius 0.15
  circle A771 centre (-5.35, 3.55) radius 0.15
  circle A772 centre (-5.35, 3.25) radius 0.15
  circle A773 centre (-5.35, 2.95) radius 0.15
  circle A774 centre (-5.35, 2.65) radius 0.15
  circle A775 centre (-5.35, 2.35) radius 0.15
  circle A776 centre (-5.35, 2.05) radius 0.15
  circle A777 centre (-5.35, 1.75) radius 0.15
  circle A778 centre (-5.35, 1.45) radius 0.15
  circle A779 centre (-5.35, 1.15) radius 0.15
  circle A780 centre (-5.35, 0.85) radius 0.15
  circle A781 centre (-5.35, 0.55) radius 0.15
  circle A782 centre (-5.35, 0.25) radius 0.15
  circle A783 centre (-5.35, -0.05) radius 0.15
  circle A784 centre (-5.35, -0.35) radius 0.15
  circle A785 centre (-5.35, -0.65) radius 0.15
  circle A786 centre (-5.35, -0.95) radius 0.15
  circle A787 centre (-5.35, -1.25) radius 0.15
  circle A788 centre (-5.35, -1.55) radius 0.15
  circle A789 centre (-5.35, -1.85) radius 0.15
  circle A790 centre (-5.35, -2.15) radius 0.15
  circle A791 centre (-5.35, -2.45) radius 0.15
  circle A792 centre (-5.35, -2.75) radius 0.15
  circle A793 centre (-5.35, -3.05) radius 0.15
  circle A794 centre (-5.35, -3.35) radius 0.15
  circle A795 centre (-5.35, -3.65) radius 0.15
  circle A796 centre (-5.35, -3.95) radius 0.15
  circle A797 centre (-5.35, -4.25) radius 0.15
  circle A798 centre (-5.35, -4.55) radius 0.15
  circle A799 centre (-5.35, -4.85) radius 0.15
  circle A800 centre (-5.05, 9.85) radius 0.15
  circle A801 centre (-5.05, 9.55) radius 0.15
  circle A802 centre (-5.05, 9.25) radius 0.15
  circle A803 centre (-5.05, 8.95) radius 0.15
  circle A804 centre (-5.05, 8.65) radius 0.15
  circle A805 centre (-5.05, 8.35) radius 0.15
  circle A806 centre (-5.05, 8.05) radius 0.15
  circle A807 centre (-5.05, 7.75) radius 0.15
  circle A808 centre (-5.05, 7.45) radius 0.15
  circle A809 centre (-5.05, 7.15) radius 0.15
  circle A810 centre (-5.05, 6.85) radius 0.15
  circle A811 centre (-5.05, 6.55) radius 0.15
  circle A812 centre (-5.05, 6.25) radius 0.15
  circle A813 centre (-5.05, 5.95) radius 0.15
  circle A814 centre (-5.05, 5.65) radius 0.15
  circle A815 centre (-5.05, 5.35) radius 0.15
  circle A816 centre (-5.05, 5.05) radius 0.15
  circle A817 centre (-5.05, 4.75) radius 0.15
  circle A818 centre (-5.05, 4.45) radius 0.15
  circle A819 centre (-5.05, 4.15) radius 0.15
  circle A820 centre (-5.05, 3.85) radius 0.15
  circle A821 centre (-5.05, 3.55) radius 0.15
  circle A822 centre (-5.05, 3.25) radius 0.15
  circle A823 centre (-5.05, 2.95) radius 0.15
  circle A824 centre (-5.05, 2.65) radius 0.15
  circle A825 centre (-5.05, 2.35) radius 0.15
  circle A826 centre (-5.05, 2.05) radius 0.15
  circle A827 centre (-5.05, 1.75) radius 0.15
  circle A828 centre (-5.05, 1.45) radius 0.15
  circle A829 centre (-5.05, 1.15) radius 0.15
  circle A830 centre (-5.05, 0.85) radius 0.15
  circle A831 centre (-5.05, 0.55) radius 0.15
  circle A832 centre (-5.05, 0.25) radius 0.15
  circle A833 centre (-5.05, -0.05) radius 0.15
  circle A834 centre (-5.05, -0.35) radius 0.15
  circle A835 centre (-5.05, -0.65) radius 0.15
  circle A836 centre (-5.05, -0.95) radius 0.15
  circle A837 centre (-5.05, -1.25) radius 0.15
  circle A838 centre (-5.05, -1.55) radius 0.15
  circle A839 centre (-5.05, -1.85) radius 0.15
  circle A840 centre (-5.05, -2.15) radius 0.15
  circle A841 centre (-5.05, -2.45) radius 0.15
  circle A842 centre (-5.05, -2.75) radius 0.15
  circle A843 centre (-5.05, -3.05) radius 0.15
  circle A844 centre (-5.05, -3.35) radius 0.15
  circle A845 centre (-5.05, -3.65) radius 0.15
  circle A846 centre (-5.05, -3.95) radius 0.15
  circle A847 centre (-5.05, -4.25) radius 0.15
  circle A848 centre (-5.05, -4.55) radius 0.15
  circle A849 centre (-5.05, -4.85) radius 0.15
  circle A850 centre (-4.75, 9.85) radius 0.15
  circle A851 centre (-4.75, 9.55) radius 0.15
  circle A852 centre (-4.75, 9.25) radius 0.15
  circle A853 centre (-4.75, 8.95) radius 0.15
  circle A854 centre (-4.75, 8.65) radius 0.15
  circle A855 centre (-4.75, 8.35) radius 0.15
  circle A856 centre (-4.75, 8.05) radius 0.15
  circle A857 centre (-4.75, 7.75) radius 0.15
  circle A858 centre (-4.75, 7.45) radius 0.15
  circle A859 centre (-4.75, 7.15) radius 0.15
  circle A860 centre (-4.75, 6.85) radius 0.15
  circle A861 centre (-4.75, 6.55) radius 0.15
  circle A862 centre (-4.75, 6.25) radius 0.15
  circle A863 centre (-4.75, 5.95) radius 0.15
  circle A864 centre (-4.75, 5.65) radius 0.15
  circle A865 centre (-4.75, 5.35) radius 0.15
  circle A866 centre (-4.75, 5.05) radius 0.15
  circle A867 centre (-4.75, 4.75) radius 0.15
  circle A868 centre (-4.75, 4.45) radius 0.15
  circle A869 centre (-4.75, 4.15) radius 0.15
  circle A870 centre (-4.75, 3.85) radius 0.15
  circle A871 centre (-4.75, 3.55) radius 0.15
  circle A872 centre (-4.75, 3.25) radius 0.15
  circle A873 centre (-4.75, 2.95) radius 0.15
  circle A874 centre (-4.75, 2.65) radius 0.15
  circle A875 centre (-4.75, 2.35) radius 0.15
  circle A876 centre (-4.75, 2.05) radius 0.15
  circle A877 centre (-4.75, 1.75) radius 0.15
  circle A878 centre (-4.75, 1.45) radius 0.15
  circle A879 centre (-4.75, 1.15) radius 0.15
  circle A880 centre (-4.75, 0.85) radius 0.15
  circle A881 centre (-4.75, 0.55) radius 0.15
  circle A882 centre (-4.75, 0.25) radius 0.15
  circle A883 centre (-4.75, -0.05) radius 0.15
  circle A884 centre (-4.75, -0.35) radius 0.15
  circle A885 centre (-4.75, -0.65) radius 0.15
  circle A886 centre (-4.75, -0.95) radius 0.15
  circle A887 centre (-4.75, -1.25) radius 0.15
  circle A888 centre (-4.75, -1.55) radius 0.15
  circle A889 centre (-4.75, -1.85) radius 0.15
  circle A890 centre (-4.75, -2.15) radius 0.15
  circle A891 centre (-4.75, -2.45) radius 0.15
  circle A892 centre (-4.75, -2.75) radius 0.15
  circle A893 centre (-4.75, -3.05) radius 0.15
  circle A894 centre (-4.75, -3.35) radius 0.15
  circle A895 centre (-4.75, -3.65) radius 0.15
  circle A896 centre (-4.75, -3.95) radius 0.15
  circle A897 centre (-4.75, -4.25) radius 0.15
  circle A898 centre (-4.75, -4.55) radius 0.15
  circle A899 centre (-4.75, -4.85) radius 0.15
  circle A900 centre (-4.45, 9.85) radius 0.15
  circle A901 centre (-4.45, 9.55) radius 0.15
  circle A902 centre (-4.45, 9.25) radius 0.15
  circle A903 centre (-4.45, 8.95) radius 0.15
  circle A904 centre (-4.45, 8.65) radius 0.15
  circle A905 centre (-4.45, 8.35) radius 0.15
  circle A906 centre (-4.45, 8.05) radius 0.15
  circle A907 centre (-4.45, 7.75) radius 0.15
  circle A908 centre (-4.45, 7.45) radius 0.15
  circle A909 centre (-4.45, 7.15) radius 0.15
  circle A910 centre (-4.45, 6.85) radius 0.15
  circle A911 centre (-4.45, 6.55) radius 0.15
  circle A912 centre (-4.45, 6.25) radius 0.15
  circle A913 centre (-4.45, 5.95) radius 0.15
  circle A914 centre (-4.45, 5.65) radius 0.15
  circle A915 centre (-4.45, 5.35) radius 0.15
  circle A916 centre (-4.45, 5.05) radius 0.15
  circle A917 centre (-4.45, 4.75) radius 0.15
  circle A918 centre (-4.45, 4.45) radius 0.15
  circle A919 centre (-4.45, 4.15) radius 0.15
  circle A920 centre (-4.45, 3.85) radius 0.15
  circle A921 centre (-4.45, 3.55) radius 0.15
  circle A922 centre (-4.45, 3.25) radius 0.15
  circle A923 centre (-4.45, 2.95) radius 0.15
  circle A924 centre (-4.45, 2.65) radius 0.15
  circle A925 centre (-4.45, 2.35) radius 0.15
  circle A926 centre (-4.45, 2.05) radius 0.15
  circle A927 centre (-4.45, 1.75) radius 0.15
  circle A928 centre (-4.45, 1.45) radius 0.15
  circle A929 centre (-4.45, 1.15) radius 0.15
  circle A930 centre (-4.45, 0.85) radius 0.15
  circle A931 centre (-4.45, 0.55) radius 0.15
  circle A932 centre (-4.45, 0.25) radius 0.15
  circle A933 centre (-4.45, -0.05) radius 0.15
  circle A934 centre (-4.45, -0.35) radius 0.15
  circle A935 centre (-4.45, -0.65) radius 0.15
  circle A936 centre (-4.45, -0.95) radius 0.15
  circle A937 centre (-4.45, -1.25) radius 0.15
  circle A938 centre (-4.45, -1.55) radius 0.15
  circle A939 centre (-4.45, -1.85) radius 0.15
  circle A940 centre (-4.45, -2.15) radius 0.15
  circle A941 centre (-4.45, -2.45) radius 0.15
  circle A942 centre (-4.45, -2.75) radius 0.15
  circle A943 centre (-4.45, -3.05) radius 0.15
  circle A944 centre (-4.45, -3.35) radius 0.15
  circle A945 centre (-4.45, -3.65) radius 0.15
  circle A946 centre (-4.45, -3.95) radius 0.15
  circle A947 centre (-4.45, -4.25) radius 0.15
  circle A948 centre (-4.45, -4.55) radius 0.15
  circle A949 centre (-4.45, -4.85) radius 0.15
  circle A950 centre (-4.15, 9.85) radius 0.15
  circle A951 centre (-4.15, 9.55) radius 0.15
  circle A952 centre (-4.15, 9.25) radius 0.15
  circle A953 centre (-4.15, 8.95) radius 0.15
  circle A954 centre (-4.15, 8.65) radius 0.15
  circle A955 centre (-4.15, 8.35) radius 0.15
  circle A956 centre (-4.15, 8.05) radius 0.15
  circle A957 centre (-4.15, 7.75) radius 0.15
  circle A958 centre (-4.15, 7.45) radius 0.15
  circle A959 centre (-4.15, 7.15) radius 0.15
  circle A960 centre (-4.15, 6.85) radius 0.15
  circle A961 centre (-4.15, 6.55) radius 0.15
  circle A962 centre (-4.15, 6.25) radius 0.15
  circle A963 centre (-4.15, 5.95) radius 0.15
  circle A964 centre (-4.15, 5.65) radius 0.15
  circle A965 centre (-4.15, 5.35) radius 0.15
  circle A966 centre (-4.15, 5.05) radius 0.15
  circle A967 centre (-4.15, 4.75) radius 0.15
  circle A968 centre (-4.15, 4.45) radius 0.15
  circle A969 centre (-4.15, 4.15) radius 0.15
  circle A970 centre (-4.15, 3.85) radius 0.15
  circle A971 centre (-4.15, 3.55) radius 0.15
  circle A972 centre (-4.15, 3.25) radius 0.15
  circle A973 centre (-4.15, 2.95) radius 0.15
  circle A974 centre (-4.15, 2.65) radius 0.15
  circle A975 centre (-4.15, 2.35) radius 0.15
  circle A976 centre (-4.15, 2.05) radius 0.15
  circle A977 centre (-4.15, 1.75) radius 0.15
  circle A978 centre (-4.15, 1.45) radius 0.15
  circle A979 centre (-4.15, 1.15) radius 0.15
  circle A980 centre (-4.15, 0.85) radius 0.15
  circle A981 centre (-4.15, 0.55) radius 0.15
  circle A982 centre (-4.15, 0.25) radius 0.15
  circle A983 centre (-4.15, -0.05) radius 0.15
  circle A984 centre (-4.15, -0.35) radius 0.15
  circle A985 centre (-4.15, -0.65) radius 0.15
  circle A986 centre (-4.15, -0.95) radius 0.15
  circle A987 centre (-4.15, -1.25) radius 0.15
  circle A988 centre (-4.15, -1.55) radius 0.15
  circle A989 centre (-4.15, -1.85) radius 0.15
  circle A990 centre (-4.15, -2.15) radius 0.15
  circle A991 centre (-4.15, -2.45) radius 0.15
  circle A992 centre (-4.15, -2.75) radius 0.15
  circle A993 centre (-4.15, -3.05) radius 0.15
  circle A994 centre (-4.15, -3.35) radius 0.15
  circle A995 centre (-4.15, -3.65) radius 0.15
  circle A996 centre (-4.15, -3.95) radius 0.15
  circle A997 centre (-4.15, -4.25) radius 0.15
  circle A998 centre (-4.15, -4.55) radius 0.15
  circle A999 centre (-4.15, -4.85) radius 0.15
  circle A1000 centre (-3.85, 9.85) radius 0.15
  circle A1001 centre (-3.85, 9.55) radius 0.15
  circle A1002 centre (-3.85, 9.25) radius 0.15
  circle A1003 centre (-3.85, 8.95) radius 0.15
  circle A1004 centre (-3.85, 8.65) radius 0.15
  circle A1005 centre (-3.85, 8.35) radius 0.15
  circle A1006 centre (-3.85, 8.05) radius 0.15
  circle A1007 centre (-3.85, 7.75) radius 0.15
  circle A1008 centre (-3.85, 7.45) radius 0.15
  circle A1009 centre (-3.85, 7.15) radius 0.15
  circle A1010 centre (-3.85, 6.85) radius 0.15
  circle A1011 centre (-3.85, 6.55) radius 0.15
  circle A1012 centre (-3.85, 6.25) radius 0.15
  circle A1013 centre (-3.85, 5.95) radius 0.15
  circle A1014 centre (-3.85, 5.65) radius 0.15
  circle A1015 centre (-3.85, 5.35) radius 0.15
  circle A1016 centre (-3.85, 5.05) radius 0.15
  circle A1017 centre (-3.85, 4.75) radius 0.15
  circle A1018 centre (-3.85, 4.45) radius 0.15
  circle A1019 centre (-3.85, 4.15) radius 0.15
  circle A1020 centre (-3.85, 3.85) radius 0.15
  circle A1021 centre (-3.85, 3.55) radius 0.15
  circle A1022 centre (-3.85, 3.25) radius 0.15
  circle A1023 centre (-3.85, 2.95) radius 0.15
  circle A1024 centre (-3.85, 2.65) radius 0.15
  circle A1025 centre (-3.85, 2.35) radius 0.15
  circle A1026 centre (-3.85, 2.05) radius 0.15
  circle A1027 centre (-3.85, 1.75) radius 0.15
  circle A1028 centre (-3.85, 1.45) radius 0.15
  circle A1029 centre (-3.85, 1.15) radius 0.15
  circle A1030 centre (-3.85, 0.85) radius 0.15
  circle A1031 centre (-3.85, 0.55) radius 0.15
  circle A1032 centre (-3.85, 0.25) radius 0.15